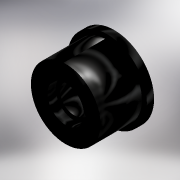
# Autodesk Inventor part: LED holder
Saved by Autodesk Inventor 2017 (Build 210142000, 142)
## iProperties
Created: 2017-03-04
Part Number: LED holder
Material: ABS Plastic
Document SubType Name: Modeling
Designer: dpgai
Density: 1.06 g/cm^3
Appearance: Black
Author: dpgai
Autodesk Inventor part; units mm, degrees
ref_plane "YZ Plane" through (0, 0, 0) normal (1, 0, 0) x (0, 1, 0)
ref_plane "XZ Plane" through (0, 0, 0) normal (0, 1, 0) x (-1, 0, 0)
ref_plane "XY Plane" through (0, 0, 0) normal (0, 0, 1) x (1, 0, 0)
sketch "Sketch1" plane through (0, 0, 0) normal (0, 0, 1) x (1, 0, 0)
  line L0 (0, 0) -> (1.65, 0)
  line L1 (1.65, 0) -> (1.65, 3)
  line L2 (1.65, 3) -> (3.6, 3)
  line L3 (3.6, 3) -> (3.6, 3.65)
  line L4 (3.6, 3.65) -> (1.65, 3.65)
  line L5 (0, 0) -> (0, 3.65)
  line L6 (1.65, 3.65) -> (0, 3.65)
  dimension "d0" = 1.65
  dimension "d1" = 1.95
  dimension "d2" = 3
  dimension "d3" = 0.65
  constraints: 14 end point, 4 perpendicular, 1 horizontal, 1 vertical
  measures "d0" distance of L0.start L0.end
  measures "d1" distance of L1.end L2.end
  measures "d2" distance of L0.end L1.end
  measures "d3" distance of L2.end L3.end
revolve "Revolution1" add sketch "Sketch1" angle 360 about axis through (0, 0, 0) along (0, 1, 0)
sketch "Sketch2" plane through (0, 0, 0) normal (1, 0, 0) x (0, 1, 0)
  line L0 (3, 1.65) -> (3, -1.65) projected
  line L1 (0, 1.65) -> (0, -1.65) projected
  line L2 (3.65, 3.6) -> (3.65, -3.6) projected
  line L3 (3, 3.6) -> (3, -3.6) projected
  line L4 (3, -1.65) -> (0, -1.65) projected
  line L5 (3, 1.65) -> (0, 1.65) projected
  line L6 (3, -3.15) -> (-0.75, -3.15)
  line L7 (-0.75, -3.15) -> (-0.75, -1.65)
  line L8 (-0.75, -1.65) -> (3, -1.65)
  line L9 (3, -1.65) -> (3, -3.15)
  line L10 (0, 0) -> (11.9884, 0)
  dimension "d5" = 3.75
  dimension "d6" = 1.5
  dimension "d12" = 3.15
  constraints: 10 end point, 2 horizontal, 2 parallel, 1 perpendicular, 1 point on line
  measures "d5" distance of L7.end L8.end
  measures "d6" distance of L6.end L7.end
  measures "d12" distance between parallel lines of L6 L10
sketch "Sketch3" plane through (0, 3.65, 0) normal (0, 1, 0) x (1, 0, 0)
  circle A0 centre (0, 0) radius 1.25
  dimension "d7" = 2.5
  constraints: 1 centre point, 1 coincident
  measures "d7" diameter of A0
revolve "Revolution2" add sketch "Sketch2" angle 360 about axis through (0, 0, 0) along (0, 1, 0) contours L3 L6 L7 L8 L4
extrude "Extrusion1" cut sketch "Sketch3" against normal through all
body "Solid1"
